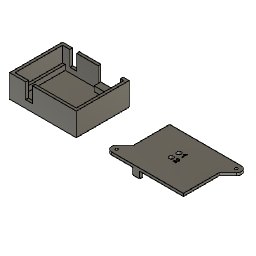
enclosure_v2 (Autodesk Fusion 360 design; units mm, degrees)
Autodesk Fusion 360 part; units mm, degrees
sketch "Sketch1" plane through (0, 0, 0) normal (0, 0, 1) x (1, 0, 0)
  line L0 (0, 0) -> (91.5, 0)
  line L1 (91.5, 0) -> (91.5, 71)
  line L2 (0, 0) -> (0, 71)
  line L3 (0, 71) -> (91.5, 71)
  line L4 (95.5, -4) -> (95.5, 75)
  line L5 (-4, 75) -> (95.5, 75)
  line L6 (-4, -4) -> (-4, 75)
  line L7 (-4, -4) -> (95.5, -4)
  line L8 (0, 0) -> (20, 0)
  line L9 (20, 0) -> (30, 0)
  line L10 (30, 0) -> (30, -4)
  line L11 (20, 0) -> (20, -4)
  line L12 (91.5, 71) -> (86.5, 71)
  line L13 (86.5, 71) -> (86.5, 75)
  line L14 (86.5, 71) -> (53, 71)
  line L15 (53, 71) -> (53, 75)
  line L16 (53, 71) -> (53, 65)
  line L17 (53, 65) -> (85, 65)
  line L18 (85, 65) -> (85, 6)
  line L19 (91.5, 0) -> (91.5, 6)
  line L20 (85, 6) -> (49.5, 6)
  line L21 (49.5, 6) -> (49.5, 0)
  line L22 (0, 0) -> (4, 0)
  line L23 (4, 0) -> (4, 71)
  line L24 (0, 71) -> (11, 71)
  line L25 (11, 71) -> (11, 75)
  line L26 (11, 71) -> (21, 71)
  line L27 (21, 71) -> (21, 75)
  line L28 (246.5, 71) -> (246.5, 75)
  line L29 (251.5, 0) -> (251.5, 71)
  line L30 (156, -4) -> (255.5, -4)
  line L31 (247.5, 6) -> (205.75, 6)
  line L32 (251.5, 0) -> (251.5, 15)
  line L33 (247.5, 15) -> (247.5, 6)
  circle A0 centre (200, 33.5) radius 3.25
  line L34 (160, 0) -> (160, 71)
  line L35 (213, 71) -> (213, 75)
  line L36 (255.5, -4) -> (255.5, 75)
  circle A1 centre (200, 45) radius 3.25
  line L37 (156, 75) -> (255.5, 75)
  line L38 (160, 0) -> (164, 0)
  line L39 (251.5, 0) -> (251.5, 6)
  line L40 (181, 71) -> (181, 75)
  line L41 (160, 0) -> (251.5, 0)
  line L42 (171, 71) -> (171, 75)
  line L43 (205.75, 6) -> (205.75, 0)
  line L44 (160, 0) -> (180, 0)
  line L45 (180, 0) -> (180, -4)
  line L46 (190, 0) -> (190, -4)
  line L47 (171, 71) -> (181, 71)
  line L48 (251.5, 15) -> (247.5, 15)
  line L49 (246.5, 67) -> (251.5, 67)
  line L50 (156, -4) -> (156, 75)
  line L51 (251.5, 71) -> (246.5, 71)
  line L52 (181, 67) -> (213, 67)
  line L53 (160, 71) -> (171, 71)
  line L54 (180, 0) -> (190, 0)
  line L55 (213, 67) -> (251.5, 67)
  line L56 (160, 71) -> (251.5, 71)
  line L57 (181, 67) -> (164, 67)
  line L58 (164, 0) -> (164, 71)
  line L59 (208.1792, 42.092) -> (207.3197, 42.0897)
  line L60 (207.3197, 42.0897) -> (207.305, 47.5664)
  spline S0 degree 2 poles (207.305, 47.5664) (206.9954, 47.2696) (206.4901, 46.9722) knots 0 0 0 1 1 1
  spline S1 degree 2 poles (206.4901, 46.9722) (205.9895, 46.6748) (205.5888, 46.5257) knots 0 0 0 1 1 1
  line L61 (205.5888, 46.5257) -> (205.5866, 47.3565)
  spline S2 degree 2 poles (205.5866, 47.3565) (206.3067, 47.6975) (206.845, 48.1812) knots 0 0 0 1 1 1
  spline S3 degree 2 poles (206.845, 48.1812) (207.3833, 48.6649) (207.6065, 49.1191) knots 0 0 0 1 1 1
  line L62 (207.6065, 49.1191) -> (208.1603, 49.1206)
  line L63 (208.1603, 49.1206) -> (208.1792, 42.092)
  line L64 (210.244, 30.9089) -> (210.2463, 30.0828)
  line L65 (210.2463, 30.0828) -> (205.6194, 30.0698)
  spline S4 degree 2 poles (205.6194, 30.0698) (205.609, 30.3802) (205.718, 30.667) knots 0 0 0 1 1 1
  spline S5 degree 2 poles (205.718, 30.667) (205.8934, 31.1402) (206.2789, 31.5996) knots 0 0 0 1 1 1
  spline S6 degree 2 poles (206.2789, 31.5996) (206.6691, 32.0591) (207.4028, 32.6628) knots 0 0 0 1 1 1
  spline S7 degree 2 poles (207.4028, 32.6628) (208.5413, 33.6019) (208.9409, 34.1474) knots 0 0 0 1 1 1
  spline S8 degree 2 poles (208.9409, 34.1474) (209.3404, 34.6976) (209.3391, 35.1846) knots 0 0 0 1 1 1
  spline S9 degree 2 poles (209.3391, 35.1846) (209.3376, 35.6956) (208.969, 36.0431) knots 0 0 0 1 1 1
  spline S10 degree 2 poles (208.969, 36.0431) (208.6051, 36.3954) (208.0178, 36.3938) knots 0 0 0 1 1 1
  spline S11 degree 2 poles (208.0178, 36.3938) (207.3971, 36.392) (207.0257, 36.0185) knots 0 0 0 1 1 1
  spline S12 degree 2 poles (207.0257, 36.0185) (206.6543, 35.645) (206.6513, 34.9861) knots 0 0 0 1 1 1
  line L66 (206.6513, 34.9861) -> (205.7677, 35.0743)
  spline S13 degree 2 poles (205.7677, 35.0743) (205.8557, 36.063) (206.4463, 36.5803) knots 0 0 0 1 1 1
  spline S14 degree 2 poles (206.4463, 36.5803) (207.0369, 37.1025) (208.0349, 37.1053) knots 0 0 0 1 1 1
  spline S15 degree 2 poles (208.0349, 37.1053) (209.0424, 37.1081) (209.6313, 36.5511) knots 0 0 0 1 1 1
  spline S16 degree 2 poles (209.6313, 36.5511) (210.2202, 35.9941) (210.2225, 35.168) knots 0 0 0 1 1 1
  spline S17 degree 2 poles (210.2225, 35.168) (210.2237, 34.7478) (210.0529, 34.3415) knots 0 0 0 1 1 1
  spline S18 degree 2 poles (210.0529, 34.3415) (209.8821, 33.9351) (209.4823, 33.4852) knots 0 0 0 1 1 1
  spline S19 degree 2 poles (209.4823, 33.4852) (209.0873, 33.0352) (208.1631, 32.2495) knots 0 0 0 1 1 1
  spline S20 degree 2 poles (208.1631, 32.2495) (207.3914, 31.598) (207.1724, 31.3634) knots 0 0 0 1 1 1
  spline S21 degree 2 poles (207.1724, 31.3634) (206.9534, 31.1336) (206.8108, 30.8992) knots 0 0 0 1 1 1
  line L67 (206.8108, 30.8992) -> (210.244, 30.9089)
  line L68 (156, -4) -> (156, 11)
  line L69 (156, -4) -> (148.5, -4)
  arc A2 (143.1967, 8.8033) -> (148.5, -4) centre (148.5, 3.5) ccw
  line L70 (143.1967, 8.8033) -> (156, 21.6066)
  line L71 (255.5, 75) -> (255.5, 60)
  line L72 (263, 75) -> (255.5, 75)
  arc A3 (268.3033, 62.1967) -> (263, 75) centre (263, 67.5) ccw
  line L73 (268.3033, 62.1967) -> (255.5, 49.3934)
  circle A4 centre (263, 67.5) radius 2
  circle A5 centre (148.5, 3.5) radius 2
  dimension "d1" = 91.5
  dimension "d3" = 71
  dimension "d16" = 79
  dimension "d17" = 99.5
  dimension "d18" = 20
  dimension "d19" = 10
  dimension "d20" = 5
  dimension "d21" = 4
  dimension "d22" = 33.5
  dimension "d24" = 42
  dimension "d25" = 4
  dimension "d34" = 11
  dimension "d35" = 10
  dimension "d83" = 91.5
  dimension "d84" = 71
  dimension "d85" = 79
  dimension "d86" = 99.5
  dimension "d87" = 20
  dimension "d88" = 10
  dimension "d89" = 5
  dimension "d90" = 4
  dimension "d91" = 33.5
  dimension "d92" = 4
  dimension "d93" = 11
  dimension "d94" = 10
  dimension "d95" = 15
  dimension "d96" = 4
  dimension "d97" = 4
  dimension "d98" = 4
  dimension "d99" = 6.5
  dimension "d100" = 6.5
  dimension "d121" = 15
  dimension "d123" = 15
  dimension "d124" = 15
  dimension "d126" = 15
  dimension "d127" = 4
  dimension "d128" = 4
  constraint coincident L0.start L2.start
  constraint horizontal L0
  constraint perpendicular L0 L1
  constraint perpendicular L0 L2
  constraint horizontal L7
  constraint horizontal L5
  constraint vertical L6
  constraint coincident L4.start L7
  constraint perpendicular L4 L7
  constraint coincident L6 L7.start
  constraint coincident L4.end L5
  constraint perpendicular L2 L8
  constraint parallel L0 L9
  constraint coincident L7 L10.end
  constraint perpendicular L7 L10
  constraint perpendicular L8 L11
  constraint perpendicular L1 L12
  constraint perpendicular L12 L13
  constraint perpendicular L13 L14
  constraint coincident L5 L15.end
  constraint perpendicular L5 L15
  constraint perpendicular L3 L16
  constraint perpendicular L1 L17
  constraint perpendicular L0 L18
  constraint perpendicular L0 L19
  constraint perpendicular L19 L20
  constraint coincident L0 L21.end
  constraint perpendicular L0 L21
  constraint perpendicular L10 L22
  constraint coincident L3 L23.end
  constraint perpendicular L3 L23
  constraint perpendicular L2 L24
  constraint coincident L5 L25.end
  constraint perpendicular L5 L25
  constraint perpendicular L25 L26
  constraint coincident L5 L27.end
  constraint perpendicular L5 L27
  constraint horizontal L41
  constraint perpendicular L29 L41
  constraint perpendicular L34 L41
  constraint horizontal L30
  constraint horizontal L37
  constraint vertical L50
  constraint coincident L36.start L30
  constraint perpendicular L30 L36
  constraint coincident L30.start L50
  constraint coincident L36.end L37
  constraint perpendicular L34 L44
  constraint parallel L41 L54
  constraint coincident L46.end L30
  constraint perpendicular L30 L46
  constraint perpendicular L44 L45
  constraint perpendicular L29 L51
  constraint perpendicular L28 L51
  constraint coincident L35.end L37
  constraint perpendicular L35 L37
  constraint perpendicular L39 L41
  constraint perpendicular L38 L46
  constraint perpendicular L34 L53
  constraint coincident L42.end L37
  constraint perpendicular L37 L42
  constraint perpendicular L42 L47
  constraint coincident L40.end L37
  constraint perpendicular L37 L40
  constraint perpendicular L29 L31
  constraint midpoint L43.end L41
  constraint perpendicular L41 L43
  constraint perpendicular L32 L41
  constraint perpendicular L29 L48
  constraint perpendicular L31 L33
  constraint coincident L58.end L53
  constraint coincident L58.end L56
  constraint coincident L49.end L29
  constraint perpendicular L29 L49
  constraint coincident L57.end L58
  constraint perpendicular L57 L58
  constraint perpendicular L30 L68
  constraint tangent L69 A2
  constraint coincident L50 L70.end
  constraint tangent A2 L70
  constraint perpendicular L37 L71
  constraint tangent L72 A3
  constraint coincident L36 L73.end
  constraint tangent A3 L73
  constraint concentric A3 A4
  constraint concentric A2 A5
  measures "d1" distance of L0.start L0.end
  measures "d3" distance of L0.start L2.end
  measures "d16" distance of L4.end L4.start
  measures "d17" distance of L4.end L5.start
  measures "d18" distance of L0.start L8.end
  measures "d19" distance of L8.end L9.end
  measures "d20" distance of L1.end L12.end
  measures "d21" distance of L12.end L13.end
  measures "d22" distance of L12.end L14.end
  measures "d24" distance of L19.end L20.end
  measures "d25" distance of L0.start L22.end
  measures "d34" distance of L2.end L24.end
  measures "d35" distance of L24.end L26.end
  measures "d83" distance of L29.start L34.start
  measures "d84" distance of L34.start L34.end
  measures "d85" distance of L30.end L36.end
  measures "d86" distance of L37.start L36.end
  measures "d87" distance of L34.start L44.end
  measures "d88" distance of L44.end L46.start
  measures "d89" distance of L28.start L29.end
  measures "d90" distance of L28.start L28.end
  measures "d91" distance of L35.start L28.start
  measures "d92" distance of L38.end L34.start
  measures "d93" distance of L42.start L34.end
  measures "d94" distance of L40.start L42.start
  measures "d95" distance of L32.end L29.start
  measures "d96" distance of L32.end L33.start
  measures "d97" distance of L52.start L40.start
  measures "d98" distance of L52.end L35.start
  measures "d99" diameter of A1
  measures "d100" diameter of A0
  measures "d121" distance of L30.start L68.end
  measures "d123" diameter of A2
  measures "d124" distance of L36.end L71.end
  measures "d126" diameter of A3
  measures "d127" diameter of A4
  measures "d128" diameter of A5
extrude "Extrude1" add sketch "Sketch1" along normal blind 7.5 contours L0 L1 L3 L12 L14 L16 L17 L18 L19 L20 L21 makes body 1
extrude "Extrude2" add sketch "Sketch1" along normal blind 7.5 separate body contours L0 L2 L3 L8 L22 L23 L24 makes body 2
extrude "Extrude3" add sketch "Sketch1" along normal blind 7.5 separate body contours L0 L7 L9 L10 L11 makes body 3
extrude "Extrude4" add sketch "Sketch1" along normal blind 7.5 contours L3 L5 L13 L14 L15 bodies 1
extrude "Extrude5" add sketch "Sketch1" along normal blind 30.5 contours L0 L1 L3 L4 L5 L7 L10 L12 L13 L19 bodies 1 3
extrude "Extrude6" add sketch "Sketch1" along normal blind 30.5 contours L3 L5 L15 L27 bodies 1
extrude "Extrude7" add sketch "Sketch1" along normal blind 7.5 contours L3 L5 L25 L26 L27 bodies 1
extrude "Extrude8" add sketch "Sketch1" along normal blind 30.5 contours L0 L2 L3 L5 L6 L7 L8 L11 L22 L24 L25 bodies 1 2
extrude "Extrude9" add sketch "Sketch1" against normal blind 4 separate body contours L0 L2 L3 L8 L22 L23 L24 | L0 L2 L3 L5 L6 L7 L8 L11 L22 L24 L25 | L0 L3 L8 L9 L16 L17 L18 L20 L21 L23 L24 L26 | L0 L7 L9 L10 L11 | L0 L1 L3 L4 L5 L7 L10 L12 L13 L19 | L3 L5 L25 L26 L27 | L0 L1 L3 L12 L14 L16 L17 L18 L19 L20 L21 | L3 L5 L15 L27 | L3 L5 L13 L14 L15 makes body 4
combine "Combine1" operation add target body 1 tool bodies 4
extrude "Extrude19" add sketch "Sketch1" against normal blind 10 separate body contours L30 L41 L45 L46 L54 makes body 5
extrude "Extrude20" add sketch "Sketch1" against normal blind 15 separate body contours L37 L40 L42 L47 L56 makes body 6
extrude "Extrude21" add sketch "Sketch1" against normal blind 4 contours L28 L35 L37 L56 | L29 L47 L49 L51 L52 L53 L55 L56 L57 L58 bodies 6
extrude "Extrude22" add sketch "Sketch1" against normal blind 4 contours L34 L38 L41 L44 L53 L56 L58 bodies 6
extrude "Extrude23" add sketch "Sketch1" against normal blind 4 separate body contours L29 L31 L32 L33 L39 L41 L43 L48 makes body 7
extrude "Extrude24" add sketch "Sketch1" along normal blind 4 contours L28 L35 L37 L56 | L28 L29 L30 L32 L36 L37 L39 L41 L46 L51 L56 L71 | L29 L47 L49 L51 L52 L53 L55 L56 L57 L58 | L35 L37 L40 L56 | L29 L31 L33 L41 L43 L44 L48 L49 L52 L54 L55 L57 L58 | L37 L40 L42 L47 L56 | L29 L31 L32 L33 L39 L41 L43 L48 | L30 L34 L37 L38 L41 L42 L44 L45 L50 L53 L56 L68 | L34 L38 L41 L44 L53 L56 L58 | L30 L41 L45 L46 L54 | L59 L60 S0 S1 L61 S2 S3 L62 L63 | L64 L65 S4 S5 S6 S7 S8 S9 S10 S11 S12 L66 S13 S14 S15 S16 S17 S18 S19 S20 S21 L67 bodies 5 6 7
extrude "Extrude25" cut sketch "Sketch1" along normal blind 5 contours L59 L60 S0 S1 L61 S2 S3 L62 L63 | L64 L65 S4 S5 S6 S7 S8 S9 S10 S11 S12 L66 S13 S14 S15 S16 S17 S18 S19 S20 S21 L67 bodies 5
extrude "Extrude26" add sketch "Sketch1" along normal blind 4 contours L36 L71 L72 A3 L73 | L50 L68 L69 A2 L70 bodies 5
named bodies: "bottom", "top"
